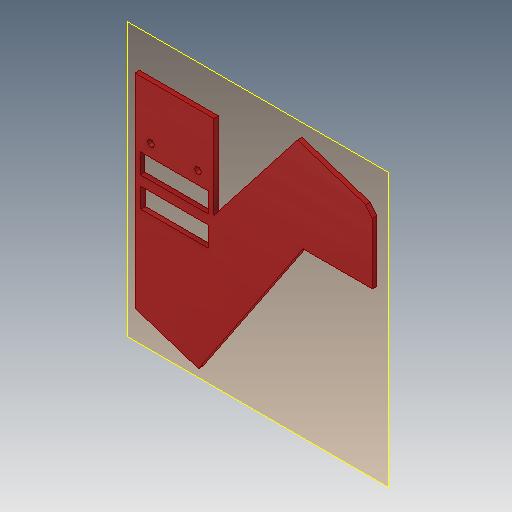
# Autodesk Inventor part: cellSTORM_v5_microscope_cover
Saved by Autodesk Inventor 2019.4 (Build 234330000, 330)
## iProperties
Created: 2020-04-27
Part Number: cellSTORM_v5_microscope_cover
Material: Generic
Document SubType Name: Modeling
Designer: diederichbenedict
Density: 1 g/cm^3
Appearance: Red
Author: diederichbenedict
Autodesk Inventor part; units mm, degrees
ref_plane "YZ Plane" through (0, 0, 0) normal (1, 0, 0) x (0, 1, 0)
ref_plane "XZ Plane" through (0, 0, 0) normal (0, 1, 0) x (-1, 0, 0)
ref_plane "XY Plane" through (0, 0, 0) normal (0, 0, 1) x (1, 0, 0)
ref_plane "Work Plane1" through (0, 0, 0) normal (0, 0, 1) x (1, 0, 0)
sketch "Sketch1" plane through (0, 0, 0) normal (0, 0, 1) x (1, 0, 0)
  circle A0 centre (-16.4512, 11.8299) radius 1.45 projected
  circle A1 centre (-37.2, 11.8299) radius 1.45 projected
  line L0 (-41.2012, 5.1624) -> (-41.2012, -2.0876) projected
  line L1 (-41.2012, -2.0876) -> (-38.2, -2.0876) projected
  line L2 (-38.2, -2.0876) -> (-38.2, -7.0876) projected
  line L3 (-38.2, -7.0876) -> (-41.2, -7.0876) projected
  line L4 (-41.2, -7.0876) -> (-41.2, -48.1342) projected
  line L5 (-41.2, -48.1342) -> (-20.7938, -54.7646) projected
  line L6 (-20.7938, -54.7646) -> (28.3237, 8.1029) projected
  line L7 (28.3237, 8.1029) -> (54.2162, 8.1029) projected
  line L8 (54.2162, 8.1029) -> (54.2162, 31.454) projected
  line L9 (54.2162, 31.454) -> (27.1735, 40.2407) projected
  line L10 (27.1735, 40.2407) -> (-12.4512, -10.4765) projected
  line L11 (-12.4512, -10.4765) -> (-12.4512, 5.6624) projected
  line L12 (-12.4512, 5.6624) -> (-15.7012, 5.6624) projected
  line L13 (-15.7012, 5.6624) -> (-15.7012, 8.1624) projected
  line L14 (-15.7012, 8.1624) -> (-12.4512, 8.1624) projected
  line L15 (-12.4512, 8.1624) -> (-12.4512, 32.1624) projected
  line L16 (-31.5338, 32.1624) -> (-41.2, 32.1624) projected
  line L17 (-41.2, 32.1624) -> (-41.2, 8.1624) projected
  line L18 (-41.2, 8.1624) -> (-38.2, 8.1624) projected
  line L19 (-38.2, 8.1624) -> (-38.2, 5.6624) projected
  line L20 (-38.2, 5.6624) -> (-41.2, 5.6624) projected
  line L21 (-41.2, 5.6624) -> (-41.2, 5.1624) projected
  line L22 (-41.2, 5.1624) -> (-41.2012, 5.1624) projected
  line L23 (-12.7012, -2.0876) -> (-12.7012, -7.0876) projected
  line L24 (-12.7012, -7.0876) -> (-15.7012, -7.0876) projected
  line L25 (-15.7012, -7.0876) -> (-15.7012, -2.0876) projected
  line L26 (-15.7012, -2.0876) -> (-12.7012, -2.0876) projected
  line L27 (-16.239, -63.6047) -> (29.7869, 5.1029) projected
  line L28 (29.7869, 5.1029) -> (60.3683, 5.1029) projected
  line L29 (60.3683, 5.1029) -> (60.3683, 31.9539) projected
  line L30 (60.3683, 31.9539) -> (57.3683, 35.6787) projected
  line L31 (57.3683, 35.6787) -> (27.4078, 45.4135) projected
  line L32 (27.4078, 45.4135) -> (-9.4512, -1.7639) projected
  line L33 (-9.4512, -1.7639) -> (-9.4512, 35.1624) projected
  line L34 (-9.4512, 35.1624) -> (-42.2, 35.1624) projected
  line L35 (-42.2, 35.1624) -> (-44.2, 35.1624) projected
  line L36 (-44.2, 35.1624) -> (-44.2, -54.5196) projected
  line L37 (-44.2, -54.5196) -> (-16.239, -63.6047) projected
  line L38 (-41.2, 5.1624) -> (-41.2, 5.6624) projected
  line L39 (-41.2, 5.6624) -> (-38.2, 5.6624) projected
  line L40 (-38.2, 5.6624) -> (-38.2, 8.1624) projected
  line L41 (-38.2, 8.1624) -> (-41.2, 8.1624) projected
  line L42 (-41.2, 8.1624) -> (-41.2, 32.1624) projected
  line L43 (-41.2, 32.1624) -> (-12.4512, 32.1624) projected
  line L44 (-12.4512, 32.1624) -> (-12.4512, 8.1624) projected
  line L45 (-12.4512, 8.1624) -> (-15.7012, 8.1624) projected
  line L46 (-15.7012, 8.1624) -> (-15.7012, 5.6624) projected
  line L47 (-15.7012, 5.6624) -> (-12.4512, 5.6624) projected
  line L48 (-12.4512, 5.6624) -> (-12.4512, -10.4765) projected
  line L49 (-12.4512, -10.4765) -> (27.1735, 40.2407) projected
  line L50 (27.1735, 40.2407) -> (54.2162, 31.454) projected
  line L51 (54.2162, 31.454) -> (54.2162, 8.1029) projected
  line L52 (54.2162, 8.1029) -> (28.3237, 8.1029) projected
  line L53 (28.3237, 8.1029) -> (-20.7938, -54.7646) projected
  line L54 (-20.7938, -54.7646) -> (-41.2, -48.1342) projected
  line L55 (-41.2, -48.1342) -> (-41.2, -7.0876) projected
  line L56 (-41.2, -7.0876) -> (-38.2, -7.0876) projected
  line L57 (-38.2, -7.0876) -> (-38.2, -2.0876) projected
  line L58 (-38.2, -2.0876) -> (-41.2012, -2.0876) projected
  line L59 (-41.2012, -2.0876) -> (-41.2012, 5.1624) projected
  line L60 (-41.2012, 5.1624) -> (-41.2, 5.1624) projected
  circle A2 centre (43.9499, 17.9141) radius 1.4 projected
  circle A3 centre (43.9499, 30.4141) radius 1.4 projected
  line L61 (-31.5338, 25.1624) -> (-31.5338, 32.1624) projected
  line L62 (-12.4512, 32.1624) -> (-22.3686, 32.1624) projected
  line L63 (-22.3686, 32.1624) -> (-22.3686, 25.1624) projected
  line L64 (-22.3686, 25.1624) -> (-31.5338, 25.1624) projected
extrude "Extrusion1" add sketch "Sketch1" along normal blind 2 contours L21 L20 L19 L18 L17 L16 L61 L64 L63 L43 L15 L14 L13 L12 L11 L10 L9 L8 L7 L6 L5 L4 L3 L2 L1 L0 | L43 L63 L64 L61 | L23 L24 L25 L26 | L37 L36 L35 L34 L33 L32 L31 L30 L29 L28 L27 | A2 | A3
sketch "Sketch4" plane through (0, 0, 2) normal (0, 0, 1) x (1, 0, 0)
  line L0 (-12.4512, -7.0876) -> (-12.4512, -15.0876) projected
  line L1 (-12.4512, -15.0876) -> (-41.2, -15.0876) projected
  line L2 (-41.2, -15.0876) -> (-41.2, -7.0876) projected
  line L3 (-41.2, -7.0876) -> (-12.4512, -7.0876) projected
  line L4 (-41.4512, -2.0876) -> (-41.4512, 5.9124) projected
  line L5 (-41.4512, 5.9124) -> (-12.4512, 5.9124) projected
  line L6 (-12.4512, 5.9124) -> (-12.4512, -2.0876) projected
  line L7 (-12.4512, -2.0876) -> (-41.4512, -2.0876) projected
  line L8 (31.1264, -1.592) -> (36.5437, 2.1484) projected
  line L9 (36.5437, 2.1484) -> (37.0695, 3.5361) projected
  line L10 (37.0695, 3.5361) -> (60.3683, 9.779) projected
  line L11 (60.3683, 9.779) -> (60.3683, 9.784) projected
  line L12 (60.3683, 9.784) -> (60.3683, 31.9539) projected
  line L13 (60.3683, 31.9539) -> (57.3683, 35.9287) projected
  line L14 (57.3683, 35.9287) -> (27.5635, 45.6128) projected
  line L15 (27.5635, 45.6128) -> (-9.4512, -1.7639) projected
  line L16 (-9.4512, -1.7639) -> (-9.4512, 35.4124) projected
  line L17 (-9.4512, 35.4124) -> (-44.2, 35.4124) projected
  line L18 (-44.2, 35.4124) -> (-44.2, -54.5196) projected
  line L19 (-44.2, -54.5196) -> (-16.239, -63.6047) projected
  line L20 (-16.239, -63.6047) -> (12.0348, -27.416) projected
  line L21 (12.0348, -27.416) -> (25.8734, -27.416) projected
  line L22 (25.8734, -27.416) -> (25.8734, -22.5432) projected
  line L23 (25.8734, -22.5432) -> (22.8734, -22.5432) projected
  line L24 (22.8734, -22.5432) -> (22.8734, -13.5432) projected
  line L25 (22.8734, -13.5432) -> (25.8734, -13.5432) projected
  line L26 (25.8734, -13.5432) -> (25.8734, 0.5361) projected
  line L27 (25.8734, 0.5361) -> (29.5751, 0.5361) projected
  line L28 (29.5751, 0.5361) -> (29.5751, -1.592) projected
  line L29 (29.5751, -1.592) -> (31.1264, -1.592) projected
  line L30 (-41.6, -6.6876) -> (-41.6, -15.4876)
  line L31 (-41.6, -15.4876) -> (-12.0512, -15.4876)
  line L32 (-12.0512, -15.4876) -> (-12.0512, -6.6876)
  line L33 (-12.0512, -6.6876) -> (-41.6, -6.6876)
  line L34 (-41.8512, 6.3124) -> (-41.8512, -2.4876)
  line L35 (-41.8512, -2.4876) -> (-12.0512, -2.4876)
  line L36 (-12.0512, -2.4876) -> (-12.0512, 6.3124)
  line L37 (-12.0512, 6.3124) -> (-41.8512, 6.3124)
  point P0 (0, 0)
  dimension "d13" = 0.4
  dimension "d14" = 0.4
  constraints: 16 end point, 6 other
  measures "d13" distance between parallel lines of L2 L30
  measures "d14" distance between parallel lines of L4 L34
extrude "Extrusion4" cut sketch "Sketch4" against normal through all contours L0 L1 L2 L3 | L4 L5 L6 L7 | L33 L32 L31 L30 | L37 L36 L35 L34
body "Solid1"
